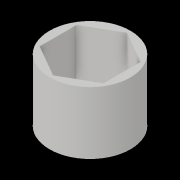
# Autodesk Inventor part: S1
Saved by Autodesk Inventor 2018 (Build 220112000, 112)
## iProperties
Created: 2022-03-31
Part Number: S1
Material: Generic
Document SubType Name: Modeling
Designer: kumpu
Density: 1 g/cm^3
Appearance: Default
Author: kumpu
## iProperties of the stored document S1_3DPrint.ipt
Created: 2022-03-31
Part Number: S1_3DPrint
Material: Generic
Document SubType Name: Modeling
Designer: kumpu
Density: 1 g/cm^3
Appearance: Default
Author: kumpu
Autodesk Inventor part; units mm, degrees
ref_plane "YZ Plane" through (0, 0, 0) normal (1, 0, 0) x (0, 1, 0)
ref_plane "XZ Plane" through (0, 0, 0) normal (0, 1, 0) x (-1, 0, 0)
ref_plane "XY Plane" through (0, 0, 0) normal (0, 0, 1) x (1, 0, 0)
sketch "Sketch1" plane through (0, 0, 0) normal (0, 1, 0) x (-1, 0, 0)
  circle A0 centre (0, 0) radius 8.255
  line L0 (-6.5405, -3.7762) -> (-6.5405, 3.7762)
  line L1 (-6.5405, 3.7762) -> (0, 7.5523)
  line L2 (0, 7.5523) -> (6.5405, 3.7762)
  line L3 (6.5405, 3.7762) -> (6.5405, -3.7762)
  line L4 (6.5405, -3.7762) -> (0, -7.5523)
  line L5 (0, -7.5523) -> (-6.5405, -3.7762)
  dimension "d0" = 16.51
  dimension "d1" = 13.081
  constraints: 12 end point, 2 coincident, 1 centre point, 1 vertical, 13 other
  measures "d0" diameter of A0
  measures "d1" distance between parallel lines of L0 L3
extrude "Extrusion1" add sketch "Sketch1" along normal blind 12.7
body "Solid1"
